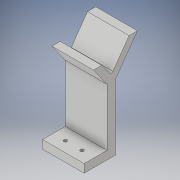
# Autodesk Inventor part: stopper
Saved by Autodesk Inventor 2019 (Build 230136000, 136)
## iProperties
Created: 2019-04-19
Part Number: stopper
Material: Generic
Document SubType Name: Modeling
Designer: Tesler
Density: 1 g/cm^3
Appearance: Default
Author: Tesler
## iProperties of the stored document stopper_3DPrint.ipt
Created: 2019-04-26
Part Number: stopper_3DPrint
Material: Generic
Document SubType Name: Modeling
Designer: Tesler
Density: 1 g/cm^3
Appearance: Default
Author: Tesler
Autodesk Inventor part; units mm, degrees
ref_plane "XZ Plane" through (0, 0, 0) normal (0, 1, 0) x (-1, 0, 0)
ref_plane "XY Plane" through (0, 0, 0) normal (0, 0, 1) x (1, 0, 0)
sketch "Sketch1" plane through (0, 0, 0) normal (1, 0, 0) x (0, 1, 0)
  line L0 (12, 4.5) -> (12, 8.5)
  line L1 (2.8235, 2) -> (12, 8.5)
  line L2 (17.8235, -12.625) -> (2.8235, -2)
  line L3 (0, 0) -> (0, 2)
  line L4 (0, 2) -> (2.8235, 2)
  line L5 (0, 0) -> (0, -2)
  line L6 (0, -2) -> (2.8235, -2)
  line L7 (12, 4.5) -> (5.6471, 0)
  line L8 (17.8235, -12.625) -> (17.8235, -8.625)
  line L9 (5.6471, 0) -> (17.8235, -8.625)
  dimension "d7" = 12
  dimension "d9" = 2
  dimension "d10" = 2
  dimension "d12" = 4
  dimension "d26" = 9.1765
  dimension "d27" = 6.3529
  dimension "d53" = 70.622
  dimension "d55" = 144.689
  dimension "d56" = 15
  constraints: 20 end point, 3 vertical, 2 perpendicular, 1 point on line
  measures "d7" distance from line of L3.start L0
  measures "d9" distance of L3.start L3.end
  measures "d10" distance of L3.start L5.end
  measures "d12" distance of L0.start L0.end
  measures "d26" horizontal distance of L1.start L0.end
  measures "d27" horizontal distance of L0.start L7.end
  measures "d53" angle of L1 L2
  measures "d55" angle of L1 L4
  measures "d56" horizontal distance of L2.start L2.end
ref_plane "Work Plane1" through (20, 0, 0) normal (1, 0, 0) x (0, 1, 0)
sketch "Sketch2" plane through (20, 0, 0) normal (1, 0, 0) x (0, 1, 0)
  line L0 (12, 4.5) -> (12, 8.5) projected
  line L1 (12, 4.5) -> (5.6471, 0) projected
  line L2 (2.8235, 2) -> (12, 8.5) projected
  line L3 (17.8235, -12.625) -> (2.8235, -2) projected
  line L4 (0, 2) -> (2.8235, 2) projected
  line L5 (0, 0) -> (0, 2) projected
  line L6 (0, 0) -> (0, -2) projected
  line L7 (0, -2) -> (2.8235, -2) projected
  line L8 (5.75, 0) -> (12, 4.5)
  line L9 (17.8235, -12.625) -> (2.8235, -2)
  line L10 (0, -2) -> (2.8235, -2)
  line L11 (0, -2) -> (0, 2)
  line L12 (0, 2) -> (2.8235, 2)
  line L13 (2.8235, 2) -> (12, 8.5)
  line L14 (12, 8.5) -> (12, 4.5)
  line L15 (17.8235, -12.625) -> (17.8235, -8.625)
  line L16 (17.8235, -8.625) -> (5.75, 0)
  dimension "d19" = 0.1029
  dimension "d57" = 4
  dimension "d58" = 71.295
  constraints: 18 end point, 4 collinear, 1 vertical
  measures "d19" distance of L1.end L8.start
  measures "d57" distance of L3.start L15.end
  measures "d58" angle of L8 L16
loft "Loft1" add profiles "Sketch1", "Sketch2"
fillet "Fillet1" radius 1 1 edges at (10, 5.6985, 0)
sketch "Sketch3" plane through (20, 0, -2) normal (1, 0, 0) x (0, 0, -1)
  line L0 (-4, 2.8235) -> (-10.5, 12) projected
  line L1 (-4, 2.8235) -> (0, 2.8235)
  line L2 (0, 2.8235) -> (0, -28.6765)
  line L3 (0, -28.6765) -> (-4, -28.6765)
  line L4 (-4, -24.6765) -> (-4, 2.8235)
  line L5 (0, -28.6765) -> (-15, -28.6765)
  line L6 (-15, -28.6765) -> (-15, -24.6765)
  line L7 (-15, -24.6765) -> (-4, -24.6765)
  line L8 (0, -24.6765) -> (0, -28.6765)
  point P0 (-2, 0)
  dimension "d35" = 31.5
  dimension "d36" = 4
  dimension "d37" = 15
  dimension "d38" = 4
  dimension "d39" = 11
  constraints: 16 end point, 4 parallel, 2 horizontal, 2 perpendicular
  measures "d35" distance between parallel lines of L1 L3
  measures "d36" distance between parallel lines of L2 L4
  measures "d37" distance of L6.end L8.start
  measures "d38" distance of L5.end L6.end
  measures "d39" distance between parallel lines of L4 L6
extrude "Extrusion2" add sketch "Sketch3" against normal up to surface (20 mm away)
sketch "Sketch4" plane through (20, -28.6765, -2) normal (0, -1, 0) x (1, 0, 0)
  line L0 (0, 15) -> (-20, 15) projected
  line L1 (-20, 0) -> (-20, 15) projected
  line L2 (0, 0) -> (0, 15) projected
  circle A0 centre (-14, 10) radius 0.7925
  circle A1 centre (-6, 10) radius 0.7925
  point P0 (-20, 2)
  dimension "d44" = 5
  dimension "d45" = 6
  dimension "d46" = 6
  dimension "d48" = 5
  dimension "d49" = 1.585
  dimension "d50" = 1.585
  constraints: 2 centre point, 2 coincident
  measures "d44" distance from line of L0 point (-14, 10)
  measures "d45" distance from line of L1 point (-14, 10)
  measures "d46" distance from line of L2 point (-6, 10)
  measures "d48" distance from line of L0 point (-6, 10)
  measures "d49" diameter of A0
  measures "d50" diameter of A1
extrude "Extrusion3" cut sketch "Sketch4" against normal blind 10
equation "\"d19\" = d15"
equation "\"d50\" = d49"
equation "\"d15\" = 0.102953"
body "Solid2"
